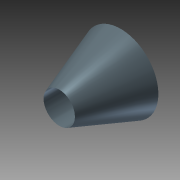
# Autodesk Inventor part: Solder Joint
Saved by Autodesk Inventor 2013 (Build 170138000, 138)
## iProperties
Created: 2013-07-31
Part Number: Solder Joint
Material: Lead
Document SubType Name: Modeling
Designer: Kyle
Density: 1 g/cm^3
Author: Kyle
Autodesk Inventor part; units mm, degrees
ref_plane "YZ Plane" through (0, 0, 0) normal (1, 0, 0) x (0, 1, 0)
ref_plane "XZ Plane" through (0, 0, 0) normal (0, 1, 0) x (-1, 0, 0)
sketch "Sketch1" plane through (0, 0, 0) normal (0, 0, 1) x (1, 0, 0)
  circle A0 centre (0, 0) radius 0.762
  line L0 (-6.3127, 2.7502) -> (-6.3127, -2.8178)
  line L1 (-6.3127, -2.8178) -> (1.3248, -2.8178)
  dimension "d0" = 1.524
  constraints: 4 end point, 1 centre point, 1 coincident, 1 perpendicular, 1 vertical
  measures "d0" diameter of A0
ref_plane "Work Plane2" through (-6.3127, -2.8178, 1.778) normal (0, 0, -1) x (1, 0, 0)
ref_plane "Work Plane1" through (-6.3127, -2.8178, 0) normal (0, 0, -1) x (1, 0, 0)
sketch "Sketch2" plane through (-6.3127, -2.8178, 1.778) normal (0, 0, -1) x (1, 0, 0)
  circle A0 centre (6.3127, -2.8178) radius 0.127
  dimension "d3" = 0.254
  constraints: 1 centre point, 1 coincident
  measures "d3" diameter of A0
loft "Loft1" add profiles "Sketch1", "Sketch2"
sketch "Sketch3" plane through (0, 0, 0) normal (0, 0, -1) x (-1, 0, 0)
  circle A0 centre (0, 0) radius 0.762 projected
  circle A1 centre (0, 0) radius 0.3175
  dimension "d9" = 0.635
  constraints: 1 centre point, 1 coincident
  measures "d9" diameter of A1
extrude "Extrusion1" cut sketch "Sketch3" against normal blind 25.4 contours A1
body "Solid1"
